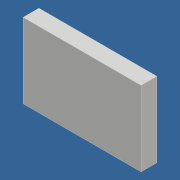
# Autodesk Inventor part: attempt
Saved by Autodesk Inventor 2017 (Build 210142000, 142)
## iProperties
Created: 2017-09-12
Part Number: attempt
Material: Generic
Document SubType Name: Modeling
Designer: Josh
Density: 1 g/cm^3
Appearance: Default
Author: Josh
Autodesk Inventor part; units mm, degrees
ref_plane "YZ Plane" through (0, 0, 0) normal (1, 0, 0) x (0, 1, 0)
ref_plane "XZ Plane" through (0, 0, 0) normal (0, 1, 0) x (-1, 0, 0)
ref_plane "XY Plane" through (0, 0, 0) normal (0, 0, 1) x (1, 0, 0)
sketch "Sketch1" plane through (0, 0, 0) normal (0, 1, 0) x (-1, 0, 0)
  line L0 (26.035, 16.51) -> (26.035, -16.51)
  line L1 (26.035, -16.51) -> (-26.035, -16.51)
  line L2 (-26.035, -16.51) -> (-26.035, 16.51)
  line L3 (-26.035, 16.51) -> (26.035, 16.51)
  point P0 (0, 0)
  point P1 (0, 0)
  dimension "d0" = 52.07
  dimension "d1" = 33.02
  constraints: 8 end point, 3 perpendicular, 2 vertical, 1 coincident, 1 horizontal
  measures "d0" distance of L0.end L1.end
  measures "d1" distance of L0.start L0.end
extrude "Extrusion1" add sketch "Sketch1" along normal blind 7
sketch "Sketch2" plane through (0, 7, 0) normal (0, 1, 0) x (1, 0, 0)
  line L0 (26.035, 16.51) -> (-26.035, 16.51) projected
  line L1 (-26.035, 16.51) -> (-26.035, -16.51) projected
  line L2 (-26.035, -16.51) -> (26.035, -16.51) projected
  line L3 (26.035, -16.51) -> (26.035, 16.51) projected
  line L4 (22.035, -12.51) -> (-22.035, -12.51)
  line L5 (-22.035, -12.51) -> (-22.035, 12.51)
  line L6 (-22.035, 12.51) -> (22.035, 12.51)
  line L7 (22.035, 12.51) -> (22.035, -12.51)
  point P0 (0, 0)
  dimension "d4" = 4
  constraints: 8 end point, 3 other
  measures "d4" distance between parallel lines of L2 L4
extrude "Extrusion2" cut sketch "Sketch2" against normal blind 4 contours L4 L5 L6 L7
body "Solid1"
